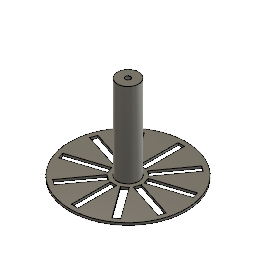
dial_column v2 (Autodesk Fusion 360 design; units mm, degrees)
Autodesk Fusion 360 part; units mm, degrees
sketch "Sketch1" plane through (0, 0, 0) normal (0, 1, 0) x (1, 0, 0)
  line L0 (-3, 15) -> (3, 15)
  line L1 (3, 15) -> (3, 55)
  line L2 (3, 55) -> (-3, 55)
  line L3 (-3, 55) -> (-3, 15)
  line L4 (8.8168, 12.1353) -> (11.2438, 10.3719)
  line L5 (8.8168, 12.1353) -> (6.3897, 13.8986)
  line L6 (6.3897, 13.8986) -> (29.9011, 46.2593)
  line L7 (29.9011, 46.2593) -> (34.7552, 42.7326)
  line L8 (34.7552, 42.7326) -> (11.2438, 10.3719)
  line L9 (14.2658, 4.6353) -> (13.3388, 7.4884)
  line L10 (13.3388, 7.4884) -> (15.1929, 1.7821)
  line L11 (15.1929, 1.7821) -> (53.2352, 14.1428)
  line L12 (53.2352, 14.1428) -> (51.3811, 19.8491)
  line L13 (51.3811, 19.8491) -> (13.3388, 7.4884)
  line L14 (14.2658, -4.6353) -> (13.3388, -7.4884)
  line L15 (13.3388, -7.4884) -> (15.1929, -1.7821)
  line L16 (15.1929, -1.7821) -> (53.2352, -14.1428)
  line L17 (53.2352, -14.1428) -> (51.3811, -19.8491)
  line L18 (51.3811, -19.8491) -> (13.3388, -7.4884)
  line L19 (8.8168, -12.1353) -> (11.2438, -10.3719)
  line L20 (11.2438, -10.3719) -> (34.7552, -42.7326)
  line L21 (34.7552, -42.7326) -> (29.9011, -46.2593)
  line L22 (29.9011, -46.2593) -> (6.3897, -13.8986)
  line L23 (6.3897, -13.8986) -> (8.8168, -12.1353)
  line L24 (0, -15) -> (3, -15)
  line L25 (3, -15) -> (-3, -15)
  line L26 (-3, -15) -> (-3, -55)
  line L27 (-3, -55) -> (3, -55)
  line L28 (3, -55) -> (3, -15)
  line L29 (-8.8168, -12.1353) -> (-6.3897, -13.8986)
  line L30 (-6.3897, -13.8986) -> (-11.2438, -10.3719)
  line L31 (-11.2438, -10.3719) -> (-34.7552, -42.7326)
  line L32 (-34.7552, -42.7326) -> (-29.9011, -46.2593)
  line L33 (-29.9011, -46.2593) -> (-6.3897, -13.8986)
  line L34 (-14.2658, -4.6353) -> (-13.3388, -7.4884)
  line L35 (-13.3388, -7.4884) -> (-15.1929, -1.7821)
  line L36 (-15.1929, -1.7821) -> (-53.2352, -14.1428)
  line L37 (-53.2352, -14.1428) -> (-51.3811, -19.8491)
  line L38 (-51.3811, -19.8491) -> (-13.3388, -7.4884)
  line L39 (-14.2658, 4.6353) -> (-13.3388, 7.4884)
  line L40 (-13.3388, 7.4884) -> (-15.1929, 1.7821)
  line L41 (-15.1929, 1.7821) -> (-53.2352, 14.1428)
  line L42 (-53.2352, 14.1428) -> (-51.3811, 19.8491)
  line L43 (-51.3811, 19.8491) -> (-13.3388, 7.4884)
  line L44 (-8.8168, 12.1353) -> (-6.3897, 13.8986)
  line L45 (-6.3897, 13.8986) -> (-11.2438, 10.3719)
  line L46 (-11.2438, 10.3719) -> (-34.7552, 42.7326)
  line L47 (-34.7552, 42.7326) -> (-29.9011, 46.2593)
  line L48 (-29.9011, 46.2593) -> (-6.3897, 13.8986)
  circle A0 centre (0, 0) radius 60
  dimension "d20" = 15
  dimension "d21" = 15
  dimension "d22" = 15
  dimension "d23" = 15
  dimension "d24" = 15
  dimension "d25" = 15
  dimension "d26" = 15
  dimension "d27" = 15
  dimension "d28" = 15
  dimension "d29" = 40
  dimension "d30" = 6
  dimension "d31" = 40
  dimension "d32" = 3
  dimension "d33" = 3
  dimension "d34" = 40
  dimension "d35" = 6
  dimension "d36" = 3
  dimension "d37" = 6
  dimension "d38" = 40
  dimension "d39" = 6
  dimension "d40" = 3
  dimension "d41" = 40
  dimension "d42" = 6
  dimension "d43" = 3
  dimension "d44" = 40
  dimension "d45" = 6
  dimension "d46" = 40
  dimension "d47" = 3
  dimension "d48" = 6
  dimension "d49" = 40
  dimension "d50" = 6
  dimension "d51" = 3
  dimension "d52" = 6
  dimension "d53" = 40
  dimension "d54" = 6
  dimension "d55" = 3
  dimension "d56" = 6
  dimension "d57" = 40
  dimension "d58" = 6
  dimension "d59" = 3
  dimension "d60" = 6
  dimension "d61" = 40
  dimension "d62" = 6
  dimension "d63" = 3
  dimension "d64" = 6
  dimension "d65" = 40
  dimension "d66" = 6
  constraint horizontal L0
  constraint perpendicular L0 L1
  constraint perpendicular L1 L2
  constraint perpendicular L2 L3
  constraint perpendicular L5 L6
  constraint perpendicular L6 L7
  constraint perpendicular L10 L11
  constraint perpendicular L11 L12
  constraint perpendicular L15 L16
  constraint perpendicular L16 L17
  constraint perpendicular L14 L18
  constraint perpendicular L19 L20
  constraint perpendicular L20 L21
  constraint perpendicular L21 L22
  constraint perpendicular L24 L26
  constraint perpendicular L26 L27
  constraint perpendicular L29 L31
  constraint perpendicular L31 L32
  constraint perpendicular L34 L36
  constraint perpendicular L36 L37
  constraint perpendicular L40 L41
  constraint perpendicular L41 L42
  constraint perpendicular L44 L46
  constraint perpendicular L46 L47
  measures "d20" distance of A0.centre L4.start
  measures "d21" distance of A0.centre L9.start
  measures "d22" distance of A0.centre L14.start
  measures "d23" distance of A0.centre L19.start
  measures "d24" distance of A0.centre L24.start
  measures "d25" distance of A0.centre L29.start
  measures "d26" distance of A0.centre L34.start
  measures "d27" distance of A0.centre L39.start
  measures "d28" distance of A0.centre L44.start
  measures "d29" distance of L0.end L1.end
  measures "d30" distance of L1.end L2.end
  measures "d31" distance of L2.end L0.start
  measures "d32" distance of L4.start L4.end
  measures "d33" distance of L4.start L5.end
  measures "d34" distance of L5.end L6.end
  measures "d35" distance of L6.end L7.end
  measures "d36" distance of L9.start L9.end
  measures "d37" distance of L9.end L10.end
  measures "d38" distance of L10.end L11.end
  measures "d39" distance of L11.end L12.end
  measures "d40" distance of L14.start L14.end
  measures "d41" distance of L15.end L16.end
  measures "d42" distance of L16.end L17.end
  measures "d43" distance of L19.start L19.end
  measures "d44" distance of L19.end L20.end
  measures "d45" distance of L20.end L21.end
  measures "d46" distance of L21.end L22.end
  measures "d47" distance of L24.start L24.end
  measures "d48" distance of L24.end L25.end
  measures "d49" distance of L25.end L26.end
  measures "d50" distance of L26.end L27.end
  measures "d51" distance of L29.start L29.end
  measures "d52" distance of L29.end L30.end
  measures "d53" distance of L30.end L31.end
  measures "d54" distance of L31.end L32.end
  measures "d55" distance of L34.start L34.end
  measures "d56" distance of L34.end L35.end
  measures "d57" distance of L35.end L36.end
  measures "d58" distance of L36.end L37.end
  measures "d59" distance of L39.start L39.end
  measures "d60" distance of L39.end L40.end
  measures "d61" distance of L40.end L41.end
  measures "d62" distance of L41.end L42.end
  measures "d63" distance of L44.start L44.end
  measures "d64" distance of L44.end L45.end
  measures "d65" distance of L45.end L46.end
  measures "d66" distance of L46.end L47.end
extrude "Extrude1" add sketch "Sketch1" along normal blind 2.5
sketch "Sketch2" plane through (0, 2.5, 0) normal (0, 1, 0) x (-1, 0, 0)
  line L0 (-11.2438, -10.3719) -> (-6.3897, -13.8986)
  line L1 (-6.3897, -13.8986) -> (-29.9011, -46.2593)
  line L2 (-29.9011, -46.2593) -> (-34.7552, -42.7326)
  line L3 (-34.7552, -42.7326) -> (-11.2438, -10.3719)
  line L4 (-29.9011, 46.2593) -> (-6.3897, 13.8986)
  line L5 (-6.3897, 13.8986) -> (-11.2438, 10.3719)
  line L6 (-11.2438, 10.3719) -> (-34.7552, 42.7326)
  line L7 (-34.7552, 42.7326) -> (-29.9011, 46.2593)
  line L8 (-3, 15) -> (-3, 55)
  line L9 (-3, 55) -> (3, 55)
  line L10 (3, 55) -> (3, 15)
  line L11 (3, 15) -> (-3, 15)
  line L12 (34.7552, -42.7326) -> (29.9011, -46.2593)
  line L13 (29.9011, -46.2593) -> (6.3897, -13.8986)
  line L14 (6.3897, -13.8986) -> (11.2438, -10.3719)
  line L15 (11.2438, -10.3719) -> (34.7552, -42.7326)
  line L16 (3, -15) -> (3, -55)
  line L17 (3, -55) -> (-3, -55)
  line L18 (-3, -55) -> (-3, -15)
  line L19 (-3, -15) -> (3, -15)
  line L20 (13.3388, 7.4884) -> (51.3811, 19.8491)
  line L21 (51.3811, 19.8491) -> (53.2352, 14.1428)
  line L22 (53.2352, 14.1428) -> (15.1929, 1.7821)
  line L23 (15.1929, 1.7821) -> (13.3388, 7.4884)
  line L24 (-13.3388, -7.4884) -> (-51.3811, -19.8491)
  line L25 (-51.3811, -19.8491) -> (-53.2352, -14.1428)
  line L26 (-53.2352, -14.1428) -> (-15.1929, -1.7821)
  line L27 (-15.1929, -1.7821) -> (-13.3388, -7.4884)
  line L28 (6.3897, 13.8986) -> (29.9011, 46.2593)
  line L29 (29.9011, 46.2593) -> (34.7552, 42.7326)
  line L30 (34.7552, 42.7326) -> (11.2438, 10.3719)
  line L31 (11.2438, 10.3719) -> (6.3897, 13.8986)
  line L32 (-53.2352, 14.1428) -> (-51.3811, 19.8491)
  line L33 (-51.3811, 19.8491) -> (-13.3388, 7.4884)
  line L34 (-13.3388, 7.4884) -> (-15.1929, 1.7821)
  line L35 (-15.1929, 1.7821) -> (-53.2352, 14.1428)
  line L36 (53.2352, -14.1428) -> (51.3811, -19.8491)
  line L37 (51.3811, -19.8491) -> (13.3388, -7.4884)
  line L38 (13.3388, -7.4884) -> (15.1929, -1.7821)
  line L39 (15.1929, -1.7821) -> (53.2352, -14.1428)
  circle A0 centre (0, 0) radius 60
  circle A1 centre (0, 0) radius 11
  dimension "d69" = 22
  constraint coincident A0.centre A1.centre
  measures "d69" diameter of A1
extrude "Extrude2" add sketch "Sketch2" along normal blind 87 contours A1
sketch "Sketch3" plane through (0, 89.5, 0) normal (0, 1, 0) x (-1, 0, 0)
  circle A0 centre (0, 0) radius 11
  arc A1 (-1.2349, 2.288) -> (1.2349, 2.288) centre (0, 0) ccw
  line L0 (1.2349, 2.288) -> (-1.2349, 2.288)
  constraint horizontal L0
extrude "Extrude3" cut sketch "Sketch3" against normal blind 30 contours A1 L0
extrude "Extrude4" cut 1 faces at (14.2269, 0.8333, -24.6855) along direction (-0.809017, 0, -0.587785) blind 0.25
extrude "Extrude5" cut 1 faces at (-3, 0.8333, -41.6667) along direction (-1, 0, 0) blind 0.25
extrude "Extrude6" cut 1 faces at (-19.081, 0.8333, -21.1588) along direction (-0.809017, 0, 0.587785) blind 0.25
extrude "Extrude7" cut 1 faces at (-27.8737, 0.8333, -5.9023) along direction (-0.309017, 0, 0.951057) blind 0.25
extrude "Extrude8" cut 1 faces at (-38.7003, 0.8333, 15.7289) along direction (0.309017, 0, 0.951057) blind 0.25
extrude "Extrude9" cut 1 faces at (-22.064, 0.8333, 35.4724) along direction (0.809017, 0, 0.587785) blind 0.25
extrude "Extrude10" cut 1 faces at (3, 0.8333, 41.6667) along direction (1, 0, 0) blind 0.25
extrude "Extrude11" cut 1 faces at (19.081, 0.8333, 21.1588) along direction (0.809017, 0, -0.587785) blind 0.25
extrude "Extrude12" cut 1 faces at (27.8737, 0.8333, 5.9023) along direction (0.309017, 0, -0.951057) blind 0.25
extrude "Extrude13" cut 1 faces at (38.7003, 0.8333, -15.7289) along direction (-0.309017, 0, -0.951057) blind 0.25
extrude "Extrude14" cut 1 faces at (27.8737, 0.8333, -5.9023) along direction (0.309017, 0, 0.951057) blind 0.25
extrude "Extrude15" cut 1 faces at (38.7003, 0.8333, 15.7289) along direction (-0.309017, 0, 0.951057) blind 0.25
extrude "Extrude16" cut 1 faces at (22.064, 0.8333, 35.4724) along direction (-0.809017, 0, 0.587785) blind 0.25
extrude "Extrude17" cut 1 faces at (-3, 0.8333, 28.3333) along direction (-1, 0, 0) blind 0.25
extrude "Extrude18" cut 1 faces at (-19.081, 0.8333, 21.1588) along direction (-0.809017, 0, -0.587785) blind 0.25
extrude "Extrude19" cut 1 faces at (-27.8737, 0.8333, 5.9023) along direction (-0.309017, 0, -0.951057) blind 0.25
extrude "Extrude20" cut 1 faces at (-38.7003, 0.8333, -15.7289) along direction (0.309017, 0, -0.951057) blind 0.25
extrude "Extrude21" cut 1 faces at (-22.064, 0.8333, -35.4724) along direction (0.809017, 0, -0.587785) blind 0.25
extrude "Extrude22" cut 1 faces at (3, 0.8333, -28.3333) along direction (1, 0, 0) blind 0.25
extrude "Extrude23" cut 1 faces at (26.9181, 0.8333, -31.9457) along direction (0.809017, 0, 0.587785) blind 0.25
